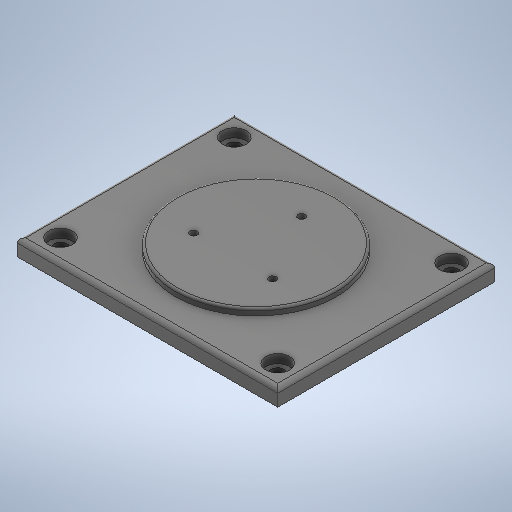
# Autodesk Inventor part: LiDAR_holder_upper
Saved by Autodesk Inventor 2026.2 (Build 302298010, 298A)
## iProperties
Created: 2026-04-16
Part Number: LiDAR_holder_upper
Material: ABS Plastic
Document SubType Name: Modeling
Designer: edi_park
Density: 1.06 g/cm^3
Appearance: Smooth - White
Author: edi_park
Autodesk Inventor part; units mm, degrees
ref_plane "YZ Plane" through (0, 0, 0) normal (1, 0, 0) x (0, 1, 0)
ref_plane "XZ Plane" through (0, 0, 0) normal (0, 1, 0) x (-1, 0, 0)
ref_plane "XY Plane" through (0, 0, 0) normal (0, 0, 1) x (1, 0, 0)
sketch "스케치1" plane through (0, 0, 0) normal (0, 1, 0) x (-1, 0, 0)
  circle A0 centre (0, 0) radius 37
  circle A1 centre (0, 0) radius 21 construction
  circle A2 centre (0, -21) radius 1.65
  circle A3 centre (18.1865, 10.5) radius 1.65
  circle A4 centre (-18.1865, 10.5) radius 1.65
  dimension "d1" = 42
  dimension "d0" = 74
  dimension "d2" = 3.3
  dimension "d6" = 360
  constraints: 4 centre point, 2 coincident, 1 vertical alignment, 9 other
  measures "d0" diameter of A0
  measures "d2" diameter of A2
extrude "돌출1" add sketch "스케치1" along normal blind 3
sketch "스케치2" plane through (0, 0, 0) normal (0, -1, 0) x (1, 0, 0)
  line L0 (60, 50) -> (-60, 50)
  line L1 (-60, 50) -> (-60, -50)
  line L2 (-60, -50) -> (60, -50)
  line L3 (60, -50) -> (60, 50)
  line L4 (60, 50) -> (-60, -50) construction
  line L5 (-60, 50) -> (60, -50) construction
  circle A0 centre (0, 0) radius 37 projected
  circle A1 centre (18.1865, 10.5) radius 1.65 projected
  circle A2 centre (-18.1865, 10.5) radius 1.65 projected
  circle A3 centre (0, -21) radius 1.65 projected
  dimension "d10" = 120
  dimension "d11" = 100
  constraints: 12 end point, 2 midpoint, 2 parallel, 1 horizontal, 1 perpendicular
  measures "d10" distance of L1.end L2.end
  measures "d11" distance of L2.end L0.start
extrude "돌출2" add sketch "스케치2" along normal blind 7.5 contours L3 L2 L1 L0 | A0
fillet "모깎기1" radius 2 4 edges at (60, 0, 0) (0, 0, -50) (-60, 0, 0) (0, 0, 50)
fillet "모깎기1" radius 1 1 edges at (37, 3, 0)
sketch "스케치5" plane through (0, -7.5, 0) normal (0, -1, 0) x (1, 0, 0)
  circle A0 centre (0, 0) radius 36 projected
extrude "돌출3" cut sketch "스케치5" against normal blind 7.5
sketch "스케치6" plane through (0, -7.5, 0) normal (0, -1, 0) x (1, 0, 0)
  circle A0 centre (-50, -40) radius 3.1
  line L0 (-60, -50) -> (60, -50) projected
  line L1 (-60, 50) -> (-60, -50) projected
  circle A1 centre (50, -40) radius 3.1
  circle A2 centre (-50, 40) radius 3.1
  circle A3 centre (50, 40) radius 3.1
  point P0 (0, 0)
  dimension "d18" = 6.2
  dimension "d19" = 10
  dimension "d20" = 10
  dimension "d21" = 120
  dimension "d22" = 100
  dimension "d25" = 100
  dimension "d32" = 80
  constraints: 4 centre point, 1 horizontal, 1 vertical, 6 other
  measures "d18" diameter of A0
  measures "d19" distance from line of A0.centre L0
  measures "d20" distance from line of A0.centre L1
  measures "d21" distance of L0.start L0.end
  measures "d22" distance of L1.start L0.start
  measures "d25" distance of A0.centre A1.centre
  measures "d32" distance of A0.centre A2.centre
extrude "돌출4" cut sketch "스케치6" against normal through all
sketch "스케치7" plane through (0, 0, 0) normal (0, 1, 0) x (1, 0, 0)
  circle A0 centre (-50, 40) radius 3.1 projected
  circle A1 centre (50, 40) radius 3.1 projected
  circle A2 centre (-50, -40) radius 3.1 projected
  circle A3 centre (50, -40) radius 3.1 projected
  circle A4 centre (0, 0) radius 37 projected
  line L0 (-58, -48) -> (-58, 48) projected
  line L1 (58, -48) -> (-58, -48) projected
  line L2 (58, 48) -> (58, -48) projected
  line L3 (-58, 48) -> (58, 48) projected
  circle A5 centre (50, -40) radius 5.5
  circle A6 centre (-50, -40) radius 5.5
  circle A7 centre (-50, 40) radius 5.5
  circle A8 centre (50, 40) radius 5.5
  dimension "d39" = 11
  dimension "d40" = 11
  dimension "d41" = 11
  dimension "d42" = 11
  constraints: 4 centre point, 4 coincident
  measures "d39" diameter of A5
  measures "d40" diameter of A6
  measures "d41" diameter of A7
  measures "d42" diameter of A8
extrude "돌출5" cut sketch "스케치7" against normal blind 4 contours A5 | A6 | A7 | A8
